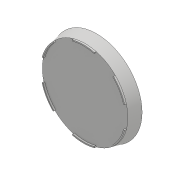
# Autodesk Inventor part: pot_holder_prototype
Saved by Autodesk Inventor 2017 (Build 210142000, 142)
## iProperties
Created: 2018-10-30
Part Number: pot_holder_prototype
Material: Generic
Document SubType Name: Modeling
Designer: mfans
Density: 1 g/cm^3
Appearance: Default
Author: mfans
Autodesk Inventor part; units mm, degrees
ref_plane "YZ Plane" through (0, 0, 0) normal (1, 0, 0) x (0, 1, 0)
ref_plane "XZ Plane" through (0, 0, 0) normal (0, 1, 0) x (-1, 0, 0)
ref_plane "XY Plane" through (0, 0, 0) normal (0, 0, 1) x (1, 0, 0)
sketch "Sketch1" plane through (0, 0, 0) normal (0, 0, 1) x (1, 0, 0)
  line L0 (0, 0) -> (37, 0)
  line L1 (37, 0) -> (39.3087, 10)
  line L2 (39.3087, 10) -> (0, 10)
  line L3 (0, 10) -> (0, 0)
  dimension "d0" = 77
  dimension "d2" = 37
  dimension "d3" = 10
  constraints: 8 end point, 1 horizontal, 1 parallel, 1 perpendicular
  measures "d0" angle of L0 L1
  measures "d2" distance of L0.start L0.end
  measures "d3" distance of L2.end L0.start
revolve "Revolution1" add sketch "Sketch1" angle 360 about axis through (0, 10, 0) along (0, -1, 0)
shell "Shell1" thickness 1.2 removed faces 1 at (-11.8053, 10, 5.6851)
fillet "Fillet1" radius 1 1 edges at (-36.0455, 1.2, 0)
sketch "Sketch2" plane through (0, 0, 0) normal (0, -1, 0) x (1, 0, 0)
  circle A0 centre (0, 0) radius 37 projected
  arc A1 (9.3175, 34.7733) -> (-9.3175, 34.7733) centre (0, 0) ccw
  line L0 (-9.3175, 34.7733) -> (-9.5763, 35.7393)
  line L1 (0, 0) -> (0, 37)
  line L2 (9.3175, 34.7733) -> (9.5763, 35.7393)
  arc A2 (9.5763, 35.7393) -> (-9.5763, 35.7393) centre (0, 0) ccw
  point P0 (0, 0)
  dimension "d8" = 72
  dimension "d9" = 15
  dimension "d10" = 15
  constraints: 7 point on circle, 6 end point, 2 centre point, 1 coincident, 1 vertical
  measures "d8" diameter of A1
  measures "d9" angle of L1 L2
  measures "d10" angle of L1 L0
extrude "Extrusion1" add sketch "Sketch2" along normal blind 1.5 contours L2 A1 L1 A0 | A0 L1 A1 L0
pattern_circular "Circular Pattern1" count 6 over 360 about axis through (0, -10, 0) along (0, 1, 0) of "Extrusion1"
body "Solid1"
